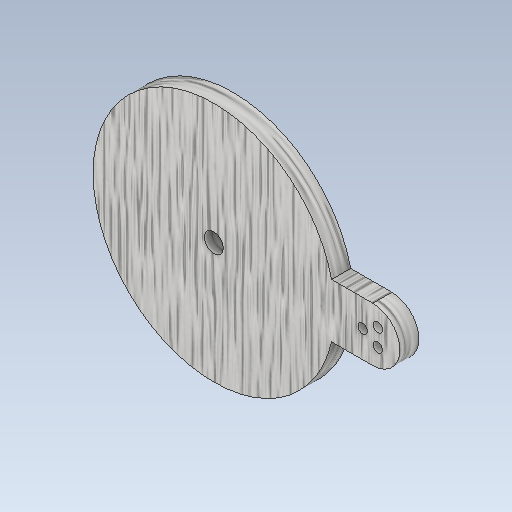
# Autodesk Inventor part: アーム最終段円盤
Saved by Autodesk Inventor 2020 (Build 240168000, 168)
## iProperties
Created: 2019-12-03
Part Number: アーム最終段円盤
Material: アルミニウム 7075
Document SubType Name: Modeling
Designer: tanjihayato
Density: 2.81 g/cm^3
Appearance: サテン - ブラシ仕上げ 重厚
Mass: 81.0965 g
Surface Area: 115.48 cm^2
Volume: 28.86 cm^3
Author: tanjihayato
Autodesk Inventor part; units mm, degrees
note: some values were not read from the file. Chosen so that the rebuilt part matches the saved one: sketch regions of "押し出し1".
ref_plane "YZ Plane" through (0, 0, 0) normal (1, 0, 0) x (0, 1, 0)
ref_plane "XZ Plane" through (0, 0, 0) normal (0, 1, 0) x (-1, 0, 0)
ref_plane "XY Plane" through (0, 0, 0) normal (0, 0, 1) x (1, 0, 0)
sketch "スケッチ1" plane through (0, 0, 0) normal (0, 0, 1) x (1, 0, 0)
  circle A0 centre (0, 0) radius 38
  line L0 (0, 0) -> (50, 0) construction
  line L1 (0, -8.5) -> (50, -8.5)
  line L2 (50, 8.5) -> (0, 8.5)
  arc A1 (0, 8.5) -> (0, -8.5) centre (0, 0) ccw
  arc A2 (50, -8.5) -> (50, 8.5) centre (50, 0) ccw
  line L3 (46.8246, 0) -> (51.5877, 2.75) construction
  line L4 (51.5877, 2.75) -> (51.5877, -2.75) construction
  line L5 (51.5877, -2.75) -> (46.8246, 0) construction
  circle A3 centre (51.5877, 2.75) radius 1.5
  circle A4 centre (46.8246, 0) radius 1.5
  circle A5 centre (51.5877, -2.75) radius 1.5
  circle A6 centre (0, 0) radius 2.995
  point P0 (25, 0)
  dimension "d0" = 76
  dimension "d2" = 50
  dimension "d3" = 17
  dimension "d4" = 3
  dimension "d5" = 3
  dimension "d6" = 3
  dimension "d7" = 5.5
  dimension "d8" = 5.99
  constraints: 14 end point, 7 centre point, 6 coincident, 4 point on circle, 4 tangent, 1 horizontal, 1 midpoint, 1 parallel, 1 point on line, 7 other
  measures "d0" diameter of A0
  measures "d2" distance of L0.start L0.end
  measures "d3" diameter of A2
  measures "d4" diameter of A3
  measures "d5" diameter of A4
  measures "d6" diameter of A5
  measures "d7" distance of L3.end L4.end
  measures "d8" diameter of A6
extrude "押し出し1" add sketch "スケッチ1" along normal blind 6
